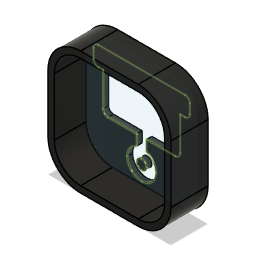
Trellis Keycap blinds (Autodesk Fusion 360 design; units mm, degrees)
Autodesk Fusion 360 part; units mm, degrees
sketch "Sketch1" plane through (0, 0, 0) normal (0, 0, 1) x (1, 0, 0)
  line L0 (2.72, 5) -> (-2.72, 5)
  line L1 (-5, 2.72) -> (-5, -2.72)
  line L2 (-2.72, -5) -> (2.72, -5)
  line L3 (5, -2.72) -> (5, 2.72)
  line L4 (5, 5) -> (-5, -5) construction
  line L5 (-5, 5) -> (5, -5) construction
  arc A0 (5, 2.72) -> (2.72, 5) centre (2.72, 2.72) ccw
  arc A1 (2.72, -5) -> (5, -2.72) centre (2.72, -2.72) ccw
  arc A2 (-5, -2.72) -> (-2.72, -5) centre (-2.72, -2.72) ccw
  arc A3 (-2.72, 5) -> (-5, 2.72) centre (-2.72, 2.72) ccw
  line L6 (-2.72, -5.2) -> (2.72, -5.2)
  arc A4 (2.72, -5.2) -> (5.2, -2.72) centre (2.72, -2.72) ccw
  line L7 (5.2, -2.72) -> (5.2, 2.72)
  arc A5 (5.2, 2.72) -> (2.72, 5.2) centre (2.72, 2.72) ccw
  line L8 (2.72, 5.2) -> (-2.72, 5.2)
  arc A6 (-2.72, 5.2) -> (-5.2, 2.72) centre (-2.72, 2.72) ccw
  line L9 (-5.2, 2.72) -> (-5.2, -2.72)
  arc A7 (-5.2, -2.72) -> (-2.72, -5.2) centre (-2.72, -2.72) ccw
  line L10 (-2.72, -5.8) -> (2.72, -5.8)
  arc A8 (2.72, -5.8) -> (5.8, -2.72) centre (2.72, -2.72) ccw
  line L11 (5.8, -2.72) -> (5.8, 2.72)
  arc A9 (5.8, 2.72) -> (2.72, 5.8) centre (2.72, 2.72) ccw
  line L12 (2.72, 5.8) -> (-2.72, 5.8)
  arc A10 (-2.72, 5.8) -> (-5.8, 2.72) centre (-2.72, 2.72) ccw
  line L13 (-5.8, 2.72) -> (-5.8, -2.72)
  arc A11 (-5.8, -2.72) -> (-2.72, -5.8) centre (-2.72, -2.72) ccw
  dimension "d1" = 10
  dimension "d2" = 10
  dimension "d3" = 2.28
  dimension "d4" = 0.2
  dimension "d5" = 0.8
  constraint horizontal L0
  constraint perpendicular L0 L1
  constraint parallel L0 L2
  constraint parallel L1 L3
  constraint coincident L4 origin
  constraint coincident L5 origin
  constraint coincident L4.start L0
  constraint coincident L4.start L3
  constraint tangent L0 A0
  constraint tangent L3 A0
  constraint coincident L5.end L3
  constraint coincident L5.end L2
  constraint tangent L3 A1
  constraint tangent L2 A1
  constraint equal A0 A1
  constraint coincident L4.end L2
  constraint coincident L4.end L1
  constraint tangent L2 A2
  constraint tangent L1 A2
  constraint equal A0 A2
  constraint coincident L5.start L1
  constraint coincident L5.start L0
  constraint tangent L1 A3
  constraint tangent L0 A3
  constraint equal A0 A3
  measures "d1" distance of L4.end L5.end
  measures "d2" distance of L5.start L4.end
  measures "d3" radius of A0
extrude "Extrude1" add sketch "Sketch1" along normal blind 3 contours L10 A8 L11 A9 L12 A10 L13 A11 makes body 1
extrude "Extrude2" add sketch "Sketch1" against normal blind 0.5 contours L0 L1 L2 L3 A0 A1 A2 A3 | L6 A4 L7 A5 L8 A6 L9 A7 | L10 A8 L11 A9 L12 A10 L13 A11 bodies 1
sketch "Sketch2" plane through (0, 0, 0) normal (0, 0, 1) x (1, 0, 0)
  line L0 (-2.72, -5.2) -> (2.72, -5.2)
  arc A0 (2.72, -5.2) -> (5.2, -2.72) centre (2.72, -2.72) ccw
  line L1 (5.2, -2.72) -> (5.2, 2.72)
  arc A1 (5.2, 2.72) -> (2.72, 5.2) centre (2.72, 2.72) ccw
  line L2 (2.72, 5.2) -> (-2.72, 5.2)
  arc A2 (-2.72, 5.2) -> (-5.2, 2.72) centre (-2.72, 2.72) ccw
  line L3 (-5.2, 2.72) -> (-5.2, -2.72)
  arc A3 (-5.2, -2.72) -> (-2.72, -5.2) centre (-2.72, -2.72) ccw
  line L4 (-4.0424, 4.14) -> (4.1303, 4.14)
  arc A4 (4.1303, 4.14) -> (4.5843, 3.6859) centre (4.1303, 3.6859) cw
  line L5 (4.5843, 3.6859) -> (4.5843, 2.7779)
  arc A5 (4.5843, 2.7779) -> (4.1303, 2.3238) centre (4.1303, 2.7779) cw
  line L6 (4.1303, 2.3238) -> (3.6763, 2.3238)
  line L7 (3.6763, 2.3238) -> (3.6763, -0.8545)
  arc A6 (3.6763, -0.8545) -> (3.2222, -1.3085) centre (3.2222, -0.8545) cw
  line L8 (3.2222, -1.3085) -> (0.498, -1.3085)
  line L9 (0.498, -1.3085) -> (0.498, -2.2938)
  spline S0 degree 3 poles (0.498, -2.2938) (1.0292, -2.4799) (1.4061, -2.9839) (1.4061, -3.5787) knots 0 0 0 0 1 1 1 1
  arc A7 (1.4061, -3.5787) -> (0.0439, -4.9408) centre (0.0439, -3.5787) cw
  arc A8 (0.0439, -4.9408) -> (-1.3182, -3.5787) centre (0.0439, -3.5787) cw
  spline S1 degree 3 poles (-1.3182, -3.5787) (-1.3182, -2.9839) (-0.9413, -2.4799) (-0.4101, -2.2938) knots 0 0 0 0 1 1 1 1
  line L10 (-0.4101, -2.2938) -> (-0.4101, -1.3085)
  line L11 (-0.4101, -1.3085) -> (-3.1344, -1.3085)
  arc A9 (-3.1344, -1.3085) -> (-3.5884, -0.8545) centre (-3.1344, -0.8545) cw
  line L12 (-3.5884, -0.8545) -> (-3.5884, 2.3238)
  line L13 (-3.5884, 2.3238) -> (-4.0424, 2.3238)
  arc A10 (-4.0424, 2.3238) -> (-4.4965, 2.7779) centre (-4.0424, 2.7779) cw
  line L14 (-4.4965, 2.7779) -> (-4.4965, 3.6859)
  arc A11 (-4.4965, 3.6859) -> (-4.0424, 4.14) centre (-4.0424, 3.6859) cw
  arc A12 (-0.4101, -3.5787) -> (0.0439, -3.1247) centre (0.0439, -3.5787) cw
  arc A13 (0.0439, -4.0328) -> (-0.4101, -3.5787) centre (0.0439, -3.5787) cw
  arc A14 (0.498, -3.5787) -> (0.0439, -4.0328) centre (0.0439, -3.5787) cw
  arc A15 (0.0439, -3.1247) -> (0.498, -3.5787) centre (0.0439, -3.5787) cw
extrude "Extrude3" cut sketch "Sketch2" against normal blind 0.5 contours L4 A4 L5 A5 L6 L7 A6 L8 L9 S0 A7 A8 S1 L10 L11 A9 L12 L13 A10 L14 A11 bodies 1 makes body 2 at (-3.1883, -3.2065, -0.5)
extrude "Extrude4" add sketch "Sketch2" against normal blind 0.5 separate body contours L4 A4 L5 A5 L6 L7 A6 L8 L9 S0 A7 A8 S1 L10 L11 A9 L12 L13 A10 L14 A11 makes body 3
named bodies: "Keycap", "Keycap (1)"
